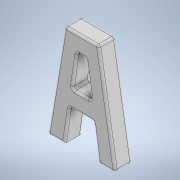
# Autodesk Inventor part: 10-18-19 C
Saved by Autodesk Inventor 2020 (Build 240168000, 168)
## iProperties
Created: 2019-10-18
Part Number: 10-18-19 C
Material: Generic
Document SubType Name: Modeling
Designer: cks4a449
Density: 1 g/cm^3
Appearance: Default
Author: cks4a449
Autodesk Inventor part; units mm, degrees
ref_plane "YZ Plane" through (0, 0, 0) normal (1, 0, 0) x (0, 1, 0)
ref_plane "XZ Plane" through (0, 0, 0) normal (0, 1, 0) x (-1, 0, 0)
ref_plane "XY Plane" through (0, 0, 0) normal (0, 0, 1) x (1, 0, 0)
sketch "Sketch1" plane through (0, 0, 0) normal (0, 0, 1) x (1, 0, 0)
  line L0 (0, 0) -> (101.6, 0)
  line L1 (50.8, 0) -> (50.8, 152.4)
  line L2 (50.8, 152.4) -> (76.2, 152.4)
  line L3 (76.2, 152.4) -> (101.6, 0)
  line L4 (50.8, 152.4) -> (25.4, 152.4)
  line L5 (25.4, 152.4) -> (0, 0)
  line L6 (50.8, 152.4) -> (50.8, 127)
  line L7 (50.8, 127) -> (57.15, 127)
  line L8 (50.8, 127) -> (44.45, 127)
  line L9 (50.8, 127) -> (50.8, 76.2)
  line L10 (50.8, 76.2) -> (88.9, 76.2)
  line L11 (50.8, 76.2) -> (12.7, 76.2)
  line L12 (50.8, 76.2) -> (50.8, 50.8)
  line L13 (50.8, 50.8) -> (93.1333, 50.8)
  line L14 (50.8, 50.8) -> (8.4667, 50.8)
  line L15 (93.1333, 50.8) -> (80.4333, 50.8)
  line L16 (88.9, 76.2) -> (76.2, 76.2)
  line L17 (12.7, 76.2) -> (25.4, 76.2)
  line L18 (8.4667, 50.8) -> (21.1667, 50.8)
  line L19 (0, 0) -> (25.4, 0)
  line L20 (101.6, 0) -> (76.2, 0)
  line L21 (44.45, 127) -> (25.4, 0)
  line L22 (57.15, 127) -> (76.2, 0)
  point P0 (36.83, 76.2)
  point P1 (64.77, 76.2)
  point P2 (68.58, 50.8)
  point P3 (33.02, 50.8)
  dimension "d0" = 101.6
  dimension "d1" = 152.4
  dimension "d2" = 25.4
  dimension "d3" = 25.4
  dimension "d4" = 25.4
  dimension "d5" = 6.35
  dimension "d6" = 6.35
  dimension "d7" = 50.8
  dimension "d8" = 25.4
  dimension "d13" = 25.4
  dimension "d14" = 25.4
  constraints: 46 end point, 11 point on line, 4 midpoint, 3 horizontal, 3 perpendicular, 1 vertical
  measures "d0" distance of L0.start L0.end
  measures "d1" distance of L1.start L1.end
  measures "d2" distance of L1.end L2.end
  measures "d3" distance of L1.end L4.end
  measures "d4" distance of L1.end L6.end
  measures "d5" distance of L6.end L7.end
  measures "d6" distance of L6.end L8.end
  measures "d7" distance of L6.end L9.end
  measures "d8" distance of L9.end L12.end
  measures "d13" distance of L0.start L19.end
  measures "d14" distance of L0.end L20.end
extrude "Extrusion1" add sketch "Sketch1" along normal blind 25.4 contours L5 L14 L21 L0 | L5 L11 L21 L14 | L21 L11 L1 L14 | L5 L4 L1 L8 L21 L11 | L22 L13 L3 L0 | L1 L10 L22 L13 | L22 L10 L3 L13 | L2 L3 L10 L22 L7 L1
fillet "Fillet1" radius 3.175 35 edges at (25.4, 152.4, 12.7) (76.2, 152.4, 12.7) (76.2, 0, 12.7) (101.6, 0, 12.7) (0, 0, 12.7) (33.02, 50.8, 12.7) (29.21, 25.4, 25.4) (12.7, 76.2, 25.4) (12.7, 76.2, 0) (59.69, 50.8, 25.4) (72.39, 25.4, 25.4) (72.39, 25.4, 0) (88.9, 76.2, 25.4) (88.9, 0, 25.4) (57.785, 76.2, 25.4) (40.64, 101.6, 25.4) (57.785, 76.2, 0) (60.96, 101.6, 25.4) (60.96, 101.6, 0) (53.975, 127, 25.4) (63.5, 152.4, 25.4) (63.5, 152.4, 0) (12.7, 0, 25.4) (59.69, 50.8, 0) (88.9, 0, 0) (12.7, 0, 0) (29.21, 25.4, 0) (68.58, 50.8, 12.7) (57.15, 127, 12.7) (53.975, 127, 0) (40.64, 101.6, 0) (64.77, 76.2, 12.7) (36.83, 76.2, 12.7) (44.45, 127, 12.7) (88.9, 76.2, 0)
body "Solid1"
